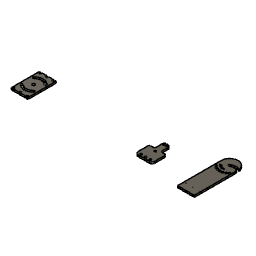
FS40 Pivot Bracket v27 (Autodesk Fusion 360 design; units mm, degrees)
Autodesk Fusion 360 part; units mm, degrees
note: some values were not read from the file. Set by a fixed rule: which sketch regions a step uses.
sketch "Schizzo5" plane through (0, 0, 0) normal (0, 0, 1) x (1, 0, 0)
  line L0 (484.2306, 82.5145) -> (484.2306, 12.5145)
  line L1 (463.4606, 82.5145) -> (463.4606, 12.5145) construction
  circle A0 centre (472.9306, 18.2645) radius 1.5
  line L2 (434.2306, 82.5145) -> (484.2306, 82.5145)
  line L3 (434.2306, 12.5145) -> (434.2306, 82.5145)
  line L4 (434.2306, 77.5145) -> (484.2306, 77.5145) construction
  circle A1 centre (463.4606, 77.5145) radius 1.5
  line L5 (472.9306, 82.5145) -> (472.9306, 12.5145) construction
  line L6 (484.2306, 12.5145) -> (434.2306, 12.5145)
  line L7 (434.2306, 18.2645) -> (484.2306, 18.2645) construction
  circle A2 centre (472.9306, 18.2645) radius 3
  circle A3 centre (463.4606, 77.5145) radius 3
  line L8 (434.2306, 47.2645) -> (484.2306, 47.2645) construction
  circle A4 centre (459.2306, 47.2645) radius 2.9
  line L9 (459.2306, 82.5145) -> (459.2306, 12.5145) construction
  circle A5 centre (459.2306, 47.2645) radius 29 construction
  line L10 (459.2306, 47.2645) -> (485, 47.2645) construction
  line L11 (459.2306, 47.2645) -> (485, 47.2645) construction
  line L12 (459.2306, 47.2645) -> (485, 47.2645) construction
  line L13 (459.2306, 47.2645) -> (485, 47.2645) construction
  circle A6 centre (459.2306, 18.2645) radius 2.9
  line L14 (631.2003, 146.4583) -> (631.2003, -8.5417)
  line L15 (581.2003, -8.5417) -> (581.2003, 146.4583)
  line L16 (631.2003, -8.5417) -> (581.2003, -8.5417)
  line L17 (610.4303, 146.4583) -> (610.4303, -8.5417) construction
  line L18 (581.2003, 146.4583) -> (631.2003, 146.4583)
  line L19 (619.9003, 146.4583) -> (619.9003, 0) construction
  line L20 (581.2003, 92.4583) -> (631.2003, 92.4583) construction
  circle A7 centre (619.9003, 92.4583) radius 1.6 construction
  line L21 (581.2003, 121.4583) -> (631.2003, 121.4583) construction
  line L22 (606.2003, 146.4583) -> (606.2003, 92.4583) construction
  circle A8 centre (606.2003, 121.4583) radius 3
  circle A9 centre (455.0006, 77.5145) radius 3
  circle A10 centre (455.0006, 77.5145) radius 1.5
  circle A11 centre (445.5306, 18.2645) radius 3
  circle A12 centre (445.5306, 18.2645) radius 1.5
  line L23 (581.2003, 96.4583) -> (631.2003, 96.4583) construction
  circle A13 centre (732, 5) radius 4
  line L24 (722, 15) -> (742, 15)
  line L25 (742, 15) -> (742, -5)
  line L26 (742, -5) -> (722, -5)
  line L27 (722, -5) -> (722, 15)
  line L28 (732, 15) -> (732, -5) construction
  line L29 (722, 5) -> (742, 5) construction
  line L30 (765, 15) -> (785, 15)
  line L31 (785, 15) -> (785, -5)
  line L32 (785, -5) -> (765, -5)
  line L33 (765, -5) -> (765, 15)
  line L34 (775, 15) -> (775, -5) construction
  line L35 (765, 5) -> (785, 5) construction
  circle A14 centre (775, 5) radius 4.05
  line L36 (606.2003, 121.4583) -> (635.9708, 121.4583) construction
  line L37 (628.1133, 97.0484) -> (631.2003, 95.2658)
  circle A15 centre (606.2003, 121.4583) radius 25
  line L38 (606.2003, 121.4583) -> (615.5972, 124.8785)
  line L39 (606.2003, 121.4583) -> (612.6158, 121.4583) construction
  line L40 (615.5972, 124.8785) -> (623.5972, 124.8785)
  line L41 (623.5972, 124.8785) -> (631.2003, 120.4889)
  line L42 (623.5972, 124.8785) -> (631.2003, 124.8785) construction
  line L43 (607.2263, 118.6393) -> (616.1262, 121.8785)
  line L44 (616.1262, 121.8785) -> (622.7934, 121.8785)
  line L45 (622.7934, 121.8785) -> (629.7003, 117.8908)
  line L46 (605.1742, 124.2774) -> (615.0682, 127.8785)
  line L47 (615.0682, 127.8785) -> (624.401, 127.8785)
  line L48 (624.401, 127.8785) -> (632.7003, 123.087)
  line L49 (629.7003, 117.8908) -> (631.2003, 117.0248)
  line L50 (629.7003, 117.8908) -> (635.1005, 117.8908) construction
  line L51 (606.2003, 121.4583) -> (598.6947, 93.4465) construction
  line L52 (606.2003, 121.4583) -> (631.0591, 121.4583) construction
  line L53 (606.2003, 121.4583) -> (629.1613, 121.4583) construction
  circle A16 centre (609.0194, 122.4844) radius 3
  circle A17 centre (476.2306, 20.5145) radius 8
  circle A18 centre (442.2306, 20.5145) radius 8
  circle A19 centre (455.0006, 77.5145) radius 5
  circle A20 centre (463.4606, 77.5145) radius 5
  line L54 (450.0006, 82.5145) -> (450.0006, 33) construction
  line L55 (434.2306, 50.1645) -> (484.2306, 50.1645) construction
  circle A21 centre (438.2296, 50.1645) radius 4
  line L56 (434.2306, 54.1645) -> (484.2306, 54.1645) construction
  circle A22 centre (446.0006, 58.1645) radius 4
  line L57 (450.0006, 77.5145) -> (450.0006, 58.1645)
  line L58 (468.4606, 77.5145) -> (468.4606, 58.1645)
  circle A23 centre (472.4606, 58.1645) radius 4
  circle A24 centre (480.2317, 50.1645) radius 4
  line L59 (438.2296, 54.1645) -> (446.0006, 54.1645)
  line L60 (480.2317, 54.1645) -> (472.4606, 54.1645)
  line L61 (606.2003, 121.4583) -> (591.7004, 96.3435) construction
  line L62 (606.2003, 121.4583) -> (625.9829, 121.4583) construction
  line L63 (606.2003, 121.4583) -> (585.6943, 100.9521) construction
  line L64 (606.2003, 121.4583) -> (623.662, 121.4583) construction
  line L65 (606.2003, 121.4583) -> (627.0131, 121.4583) construction
  line L66 (605.0102, 102.4865) -> (609.02, 102.527) construction
  line L67 (609.02, 102.527) -> (608.9899, 105.5135) construction
  line L68 (608.9899, 105.5135) -> (604.98, 105.473) construction
  line L69 (604.98, 105.473) -> (605.0102, 102.4865) construction
  line L70 (609.6489, 101.3799) -> (612.6489, 101.3799) construction
  line L71 (612.6489, 101.3799) -> (612.6489, 105.3799) construction
  line L72 (612.6489, 105.3799) -> (609.6489, 105.3799) construction
  line L73 (609.6489, 105.3799) -> (609.6489, 101.3799) construction
  line L74 (615.0517, 103.2642) -> (619.0517, 103.2642) construction
  line L75 (619.0517, 103.2642) -> (619.0517, 108.2642) construction
  line L76 (619.0517, 108.2642) -> (615.0517, 108.2642) construction
  line L77 (615.0517, 108.2642) -> (615.0517, 103.2642) construction
  line L78 (619.5121, 109.488) -> (622.5272, 109.5277) construction
  line L79 (622.5272, 109.5277) -> (622.4879, 112.512) construction
  line L80 (622.4879, 112.512) -> (619.4728, 112.4723) construction
  line L81 (619.4728, 112.4723) -> (619.5121, 109.488) construction
  line L82 (80.7173, 80.3147) -> (80.7173, -3.6853)
  circle A25 centre (85.7173, -1.1853) radius 1.5
  circle A26 centre (105.7173, 38.3147) radius 25 construction
  arc A27 (125.5163, 58.1137) -> (105.7173, 66.3147) centre (105.7173, 38.3147) ccw
  circle A28 centre (123.395, 55.9924) radius 3
  circle A29 centre (88.0397, 55.9924) radius 3
  arc A30 (105.7173, 66.3147) -> (85.9183, 58.1137) centre (105.7173, 38.3147) ccw
  circle A31 centre (125.7173, 77.8147) radius 3
  arc A32 (105.7173, 10.3147) -> (125.5163, 18.5157) centre (105.7173, 38.3147) ccw
  line L83 (80.7173, 38.3147) -> (130.7173, 38.3147) construction
  circle A33 centre (105.7173, 77.8147) radius 1.5
  circle A34 centre (85.7173, 77.8147) radius 3
  line L84 (105.7173, 38.3147) -> (123.395, 20.6371) construction
  arc A35 (105.7173, 66.3147) -> (85.9183, 58.1137) centre (105.7173, 38.3147) ccw
  circle A36 centre (85.7173, 77.8147) radius 1.5
  line L85 (130.7173, 80.3147) -> (80.7173, 80.3147)
  arc A37 (125.5163, 58.1137) -> (105.7173, 66.3147) centre (105.7173, 38.3147) ccw
  circle A38 centre (125.7173, 77.8147) radius 1.5
  line L86 (105.7173, 38.3147) -> (89.6274, 54.4047) construction
  circle A39 centre (105.7173, 77.8147) radius 3
  arc A40 (105.7173, 10.3147) -> (125.5163, 18.5157) centre (105.7173, 38.3147) ccw
  line L87 (105.7173, 38.3147) -> (105.7173, 13.3147) construction
  circle A41 centre (105.7173, 38.3147) radius 4
  circle A42 centre (105.7173, -1.1853) radius 1.5
  circle A43 centre (88.0397, 20.6371) radius 3
  line L88 (130.7173, -3.6853) -> (130.7173, 80.3147)
  arc A44 (85.9183, 18.5157) -> (105.7173, 10.3147) centre (105.7173, 38.3147) ccw
  line L89 (85.7173, 80.3147) -> (85.7173, -3.6853) construction
  arc A45 (105.7173, 13.3147) -> (123.395, 20.6371) centre (105.7173, 38.3147) ccw
  circle A46 centre (123.395, 20.6371) radius 3
  circle A47 centre (85.7173, -1.1853) radius 3
  circle A48 centre (105.7173, -1.1853) radius 3
  circle A49 centre (125.7173, -1.1853) radius 1.5
  line L90 (105.7173, 38.3147) -> (123.668, 56.2654) construction
  line L91 (80.7173, -3.6853) -> (130.7173, -3.6853)
  circle A50 centre (125.7173, -1.1853) radius 3
  line L92 (80.7173, -1.1853) -> (130.7173, -1.1853) construction
  line L93 (105.7173, 38.3147) -> (88.0397, 20.6371) construction
  arc A51 (85.9183, 18.5157) -> (105.7173, 10.3147) centre (105.7173, 38.3147) ccw
  line L94 (105.7173, 80.3147) -> (105.7173, -3.6853) construction
  arc A52 (88.0397, 20.6371) -> (105.7173, 13.3147) centre (105.7173, 38.3147) ccw
  line L95 (105.7173, 38.3147) -> (105.7173, 63.3147) construction
  line L96 (105.7173, 38.3147) -> (105.7173, 63.3147) construction
  line L97 (105.7173, 38.3147) -> (105.7173, 13.3147) construction
  circle A53 centre (606.2003, 121.4583) radius 29 construction
  line L98 (606.2003, 121.4583) -> (606.2003, 92.4583) construction
  circle A54 centre (585.6943, 100.9521) radius 3
  circle A55 centre (591.7004, 96.3435) radius 3
  circle A56 centre (598.6947, 93.4465) radius 3
  circle A57 centre (606.2003, 92.4583) radius 3
  circle A58 centre (613.7059, 93.4465) radius 3
  circle A59 centre (620.7001, 96.3435) radius 3
  circle A60 centre (626.7062, 100.9521) radius 3
  circle A61 centre (619.9003, 92.4583) radius 3 construction
  arc A62 (105.7173, 16.3147) -> (121.2737, 22.7584) centre (105.7173, 38.3147) ccw
  arc A63 (90.161, 22.7584) -> (105.7173, 16.3147) centre (105.7173, 38.3147) ccw
  arc A64 (105.7173, 60.3147) -> (90.161, 53.8711) centre (105.7173, 38.3147) ccw
  arc A65 (121.2737, 53.8711) -> (105.7173, 60.3147) centre (105.7173, 38.3147) ccw
  dimension "d70" = 50
  dimension "d71" = 70
  dimension "d72" = 29.23
  dimension "d73" = 38.7
  dimension "d74" = 59.25
  dimension "d75" = 5
  dimension "d76" = 3
  dimension "d77" = 3
  dimension "d78" = 6
  dimension "d79" = 6
  dimension "d84" = 29
  dimension "d85" = 5.8
  dimension "d103" = 5.8
  dimension "d110" = 50
  dimension "d111" = 155
  dimension "d112" = 29.23
  dimension "d113" = 38.7
  dimension "d117" = 3.2
  dimension "d119" = 29
  dimension "d120" = 6
  dimension "d129" = 6
  dimension "d130" = 3
  dimension "d131" = 29.23
  dimension "d132" = 6
  dimension "d133" = 3
  dimension "d135" = 38.7
  dimension "d137" = 25
  dimension "d139" = 8
  dimension "d145" = 20
  dimension "d146" = 20
  dimension "d152" = 20
  dimension "d153" = 20
  dimension "d154" = 8.1
  dimension "d168" = 20
  dimension "d169" = 8
  dimension "d170" = 30
  dimension "d175" = 10
  dimension "d176" = 3
  dimension "d177" = -3
  dimension "d178" = 30
  dimension "d187" = 8
  dimension "d188" = 8
  dimension "d189" = 4
  dimension "d196" = 15
  dimension "d197" = 15
  dimension "d198" = 15
  dimension "d202" = 130
  dimension "d212" = 3
  dimension "d215" = 3
  dimension "d216" = 3
  dimension "d217" = 3
  dimension "d219" = 3
  dimension "d220" = 3
  dimension "d221" = 50
  dimension "d222" = 84
  dimension "d223" = 2.5
  dimension "d224" = 20
  dimension "d225" = 3
  dimension "d226" = 6
  dimension "d227" = 3
  dimension "d228" = 6
  dimension "d229" = 8
  dimension "d230" = 45
  dimension "d231" = 6
  dimension "d232" = 45
  dimension "d233" = 6
  dimension "d238" = 58
  dimension "d239" = 6
  dimension "d240" = 6
  dimension "d241" = 6
  dimension "d242" = 6
  dimension "d243" = 6
  dimension "d245" = 58
  dimension "d246" = -3
  dimension "d247" = -3
  text T0 "0°" font "Arial" height 3 align left top in box 4.01 x 2.9866 at (605.0102, 102.4865) x (0.999949, 0.010082) y (-0.010082, 0.999949) spacing 1
  text T1 "15°" font "Arial" height 3 align left top in box 3 x 4 at (609.6489, 101.3799) x (1, 0) y (0, 1) spacing 1
  text T2 "30°" font "Arial" height 3 align left top in box 4 x 5 at (615.0517, 103.2642) x (1, 0) y (0, 1) spacing 1
  text T3 "45°" font "Arial" height 3 align left top in box 3.0153 x 2.9846 at (619.5121, 109.488) x (0.999913, 0.01317) y (-0.01317, 0.999913) spacing 1
  constraint horizontal L6
  constraint vertical L3
  constraint horizontal L2
  constraint vertical L0
  constraint coincident L1.start L2
  constraint coincident L1.end L6
  constraint perpendicular L1 L6
  constraint coincident L5.start L2
  constraint perpendicular L2 L5
  constraint coincident L4.start L3
  constraint coincident L4.end L0
  constraint perpendicular L0 L4
  constraint coincident L7.start L3
  constraint coincident L7.end L0
  constraint perpendicular L0 L7
  constraint coincident A1.centre L1
  constraint coincident A1.centre L4
  constraint coincident A0.centre L5
  constraint coincident A0.centre L7
  constraint concentric A0 A2
  constraint concentric A1 A3
  constraint coincident L3 L8.start
  constraint coincident L0 L8.end
  constraint perpendicular L0 L8
  constraint midpoint L2 L9.start
  constraint midpoint L6 L9.end
  constraint coincident A4.centre L9
  constraint coincident L8 A4.centre
  constraint concentric A4 A5
  constraint horizontal L10
  constraint coincident A4.centre A5.centre
  constraint horizontal L11
  constraint horizontal L12
  constraint horizontal L13
  constraint coincident A5 A6.centre
  constraint coincident L9 A6.centre
  constraint horizontal L16
  constraint vertical L15
  constraint horizontal L18
  constraint vertical L14
  constraint coincident L17.start L18
  constraint coincident L17.end L16
  constraint perpendicular L16 L17
  constraint coincident L19.start L18
  constraint perpendicular L18 L19
  constraint coincident L20.start L15
  constraint coincident L20.end L14
  constraint perpendicular L14 L20
  constraint coincident A7.centre L19
  constraint coincident A7.centre L20
  constraint coincident L15 L21.start
  constraint coincident L14 L21.end
  constraint perpendicular L14 L21
  constraint midpoint L18 L22.start
  constraint midpoint L20 L22.end
  constraint midpoint L21 A8.centre
  constraint coincident L4 A9.centre
  constraint concentric A9 A10
  constraint coincident L7 A11.centre
  constraint concentric A11 A12
  constraint coincident L15 L23.start
  constraint coincident L14 L23.end
  constraint perpendicular L14 L23
  constraint horizontal L24
  constraint vertical L25
  constraint horizontal L26
  constraint vertical L27
  constraint midpoint L24 L28.start
  constraint midpoint L26 L28.end
  constraint midpoint L27 L29.start
  constraint midpoint L25 L29.end
  constraint coincident A13.centre L28
  constraint coincident A13.centre L29
  constraint horizontal L30
  constraint vertical L31
  constraint horizontal L32
  constraint vertical L33
  constraint midpoint L30 L34.start
  constraint midpoint L32 L34.end
  constraint midpoint L33 L35.start
  constraint midpoint L31 L35.end
  constraint midpoint L34 A14.centre
  constraint horizontal L36
  constraint coincident A8.centre L36.start
  constraint coincident L14 L37.end
  constraint tangent L15 A15
  constraint tangent L18 A15
  constraint tangent L14 A15
  constraint horizontal L39
  constraint horizontal L40
  constraint horizontal L42
  constraint coincident L14 L41.end
  constraint horizontal L50
  constraint coincident L14 L49.end
  constraint horizontal L52
  constraint horizontal L53
  constraint coincident A8 A16.centre
  constraint coincident L38 A16.centre
  constraint coincident A8.centre A16
  constraint coincident L14 L42.end
  constraint tangent L6 A17
  constraint tangent L0 A17
  constraint symmetric L9 A17 A18
  constraint concentric A9 A19
  constraint tangent L2 A19
  constraint symmetric L9 A19 A20
  constraint coincident L2 L54.start
  constraint perpendicular L8 L54
  constraint tangent A19 L54
  constraint coincident L3 L55.start
  constraint coincident L0 L55.end
  constraint perpendicular L0 L55
  constraint tangent A4 L55
  constraint coincident L55 A21.centre
  constraint coincident L3 L56.start
  constraint coincident L0 L56.end
  constraint perpendicular L0 L56
  constraint tangent A21 L56
  constraint tangent L56 A22
  constraint tangent L54 A22
  constraint coincident A19 L57.start
  constraint coincident A22 L57.end
  constraint coincident L54 L57.end
  constraint symmetric L9 A21 A24
  constraint symmetric L9 A22 A23
  constraint symmetric L9 L57.start L58.start
  constraint symmetric L9 L57.end L58.end
  constraint coincident L56 L59.start
  constraint coincident A21 L59.start
  constraint coincident A22 L59.end
  constraint coincident L56 L59.end
  constraint symmetric L9 L59.start L60.start
  constraint symmetric L9 L59.end L60.end
  constraint tangent A19 L57
  constraint horizontal L62
  constraint horizontal L64
  constraint horizontal L65
  constraint coincident L5.end L6
  constraint horizontal L91
  constraint vertical L88
  constraint horizontal L85
  constraint vertical L82
  constraint midpoint L94.start L85
  constraint midpoint L94.end L91
  constraint coincident L92.end L88
  constraint perpendicular L88 L92
  constraint midpoint L83.start L82
  constraint midpoint L83.end L88
  constraint coincident L89.start L85
  constraint coincident L89.end L91
  constraint perpendicular L89 L91
  constraint coincident A25.centre L92
  constraint coincident A25.centre L89
  constraint concentric A25 A47
  constraint symmetric A25 A49 L94
  constraint symmetric A47 A50 L94
  constraint symmetric A25 L83 A36
  constraint symmetric L83 A34 A47
  constraint symmetric L83 A38 A49
  constraint symmetric A31 L83 A50
  constraint coincident A42.centre L94
  constraint coincident A42.centre L92
  constraint concentric A42 A48
  constraint symmetric L83 A33 A42
  constraint symmetric L83 A39 A48
  constraint midpoint A26.centre L83
  constraint concentric A26 A41
  constraint tangent A26 L88
  constraint coincident L87.end A26
  constraint coincident L87.end L94
  constraint coincident A26.centre A27.centre
  constraint coincident A43.centre L93.end
  constraint coincident L84.end A45.end
  constraint coincident L95.end A26
  constraint coincident L95.end L94
  constraint symmetric A29 L83 A43
  constraint symmetric A28 L83 A46
  constraint symmetric A32.start A27.end L83
  constraint symmetric A44.start A30.end L83
  constraint symmetric A30 L83 A44
  constraint symmetric A32.end A27.start L83
  constraint symmetric A27 L83 A40
  constraint symmetric A30.end A44.start L83
  constraint symmetric L83 A35 A51
  constraint symmetric A32 L83 A37
  constraint coincident L63.end A53
  constraint coincident A53 L22.end
  constraint perpendicular L52 L98
  constraint coincident L61.end A53
  constraint coincident L51.end A53
  constraint coincident L63.end A54.centre
  constraint coincident L61.end A55.centre
  constraint coincident L51.end A56.centre
  constraint coincident L22.end L98.end
  constraint symmetric L98 A54 A60
  constraint symmetric L98 A55 A59
  constraint symmetric L98 A56 A58
  constraint concentric A7 A61
  constraint symmetric L83 A62.end A65.start
  constraint symmetric L83 A62.start A64.start
  constraint symmetric L83 A62 A65
  constraint symmetric L83 A63.start A64.end
  constraint symmetric L83 A63 A64
  constraint coincident L92.start L82
  measures "d70" distance of L3.start L0.end
  measures "d71" distance of L0.end L0.start
  measures "d72" distance of L1 L3
  measures "d73" distance of L3 L5
  measures "d74" distance of L4 L7
  measures "d75" distance of L2 L4
  measures "d76" diameter of A1
  measures "d77" diameter of A0
  measures "d78" diameter of A2
  measures "d79" diameter of A3
  measures "d84" distance of L7 L8
  measures "d85" diameter of A4
  measures "d103" diameter of A6
  measures "d110" distance of L14.end L15.start
  measures "d111" distance of L14.end L14.start
  measures "d112" distance of L15 L17
  measures "d113" distance of L15 L19
  measures "d117" diameter of A7
  measures "d119" distance of L20 L21
  measures "d120" diameter of A8
  measures "d129" diameter of A9
  measures "d130" diameter of A10
  measures "d131" distance of L0 A9.centre
  measures "d132" diameter of A11
  measures "d133" diameter of A12
  measures "d135" distance of L0 A11.centre
  measures "d137" distance of L21 L23
  measures "d139" diameter of A13
  measures "d145" distance of L24.start L24.end
  measures "d146" distance of L24.start L26.end
  measures "d152" distance of L30.start L30.end
  measures "d153" distance of L30.start L32.end
  measures "d154" diameter of A14
  measures "d168" angle of L38 L39
  measures "d169" distance of L38.end L40.end
  measures "d170" angle of L41 L42
  measures "d175" distance of A8.centre L38.end
  measures "d178" angle of L49 L50
  measures "d187" radius of A17
  measures "d188" diameter of A21
  measures "d189" radius of A22
  measures "d196" angle of L61 L63
  measures "d197" angle of L51 L61
  measures "d198" angle of L22 L51
  measures "d202" distance of L16 L21
  measures "d221" distance of L82.end L88.start
  measures "d222" distance of L82.end L82.start
  measures "d223" distance of L91 L92
  measures "d224" distance of L89 L94
  measures "d225" diameter of A25
  measures "d226" diameter of A47
  measures "d227" diameter of A42
  measures "d228" diameter of A48
  measures "d229" diameter of A41
  measures "d230" angle of L93 L97
  measures "d231" diameter of A43
  measures "d232" angle of L84 L87
  measures "d233" diameter of A46
  measures "d238" diameter of A53
  measures "d239" diameter of A54
  measures "d240" diameter of A55
  measures "d241" diameter of A56
  measures "d242" diameter of A57
  measures "d243" diameter of A61
  measures "d245" diameter of A5
extrude "Estrusione12" add sketch "Schizzo5" along normal blind 5 contours A24 | L0 L3 L6 A17 A18 A19 A20 A21 A22 L57 L58 A23 A24 L59 L60 | L2 A19 A20 | A19 A20 | A17 | A19 A20 | A19 A20 | A18 | A21 makes body 1
extrude "Estrusione13" add sketch "Schizzo5" along normal blind 1.8 contours A2 | A3 | A9 | A11 bodies 1
extrude "Estrusione24" add sketch "Schizzo5" along normal blind 5 separate body contours L82 A31 A34 L85 A39 L88 A47 A48 L91 A50 makes body 2
extrude "Estrusione25" add sketch "Schizzo5" along normal blind 1.8 contours A34 L85 | A47 L91 | L85 A39 | A48 L91 | A31 L85 | L91 A50 picked at (85.7547, 79.98) picked at (85.7547, -3.3505) picked at (105.7547, 79.98) picked at (105.7547, -3.3505) picked at (125.7547, 79.98) picked at (125.7547, -3.3505) bodies 2
extrude "Estrusione15" add sketch "Schizzo5" along normal blind 5 separate body contours A8 A15 L43 L44 L45 L46 L47 L48 L49 | L14 L15 L16 A15 L49 | A8 L46 A16 | A8 L43 A16 makes body 3
sketch "Foratura Spalla" plane through (0, -8.5417, 0) normal (0, -1, 0) x (1, 0, 0)
  line L0 (581.2003, 0) -> (631.2003, 0)
  line L1 (631.2003, 0) -> (631.2003, 5)
  line L2 (631.2003, 5) -> (581.2003, 5)
  line L3 (581.2003, 5) -> (581.2003, 0)
  line L4 (581.2003, 2.5) -> (631.2003, 2.5) construction
  line L5 (606.2003, 5) -> (606.2003, 0) construction
  circle A0 centre (606.2003, 2.5) radius 1.4
  line L6 (586.2003, 0) -> (586.2003, 5) construction
  circle A1 centre (586.2003, 2.5) radius 1.4
  circle A2 centre (626.2003, 2.5) radius 1.4
  dimension "d124" = 2.8
  dimension "d125" = 20
  dimension "d126" = 2.8
  constraint midpoint L3 L4.start
  constraint midpoint L1 L4.end
  constraint midpoint L2 L5.start
  constraint midpoint L0 L5.end
  constraint midpoint L5 A0.centre
  constraint coincident L0 L6.start
  constraint coincident L2 L6.end
  constraint perpendicular L2 L6
  constraint midpoint L6 A1.centre
  constraint symmetric L5 A1 A2
  measures "d124" diameter of A0
  measures "d125" distance of A0.centre L6
  measures "d126" diameter of A1
extrude "Estrusione16" cut sketch "Foratura Spalla" against normal blind 20 contours A0 | A1 | A2 bodies 3
extrude "Estrusione17" add sketch "Schizzo5" along normal blind 5 separate body contours A13 makes body 4
sketch "Schizzo15" plane through (0, 0, 5) normal (0, 0, 1) x (-1, 0, 0)
  line L0 (-607.9933, -125.3035) -> (-615.0682, -127.8785)
  line L1 (-615.0682, -127.8785) -> (-624.401, -127.8785)
  line L2 (-624.401, -127.8785) -> (-631.0677, -124.0296)
  arc A0 (-631.0677, -124.0296) -> (-581.2003, -121.4583) centre (-606.2003, -121.4583) ccw
  line L3 (-581.2003, -121.4583) -> (-581.2003, 8.5417)
  line L4 (-581.2003, 8.5417) -> (-631.2003, 8.5417)
  line L5 (-631.2003, 8.5417) -> (-631.2003, -117.0248)
  line L6 (-631.2003, -117.0248) -> (-622.7934, -121.8785)
  line L7 (-622.7934, -121.8785) -> (-616.1262, -121.8785)
  line L8 (-616.1262, -121.8785) -> (-610.0454, -119.6653)
  arc A1 (-608.4984, -119.53) -> (-610.0454, -119.6653) centre (-609.0194, -122.4844) ccw
  arc A2 (-606.7212, -124.4128) -> (-608.4984, -119.53) centre (-606.2003, -121.4583) ccw
  arc A3 (-607.9933, -125.3035) -> (-606.7212, -124.4128) centre (-609.0194, -122.4844) ccw
  line L9 (-604.6879, -101.2309) -> (-607.7132, -101.231) construction
  line L10 (-607.7132, -101.231) -> (-607.713, -104.9906) construction
  line L11 (-607.713, -104.9906) -> (-604.6877, -104.9904) construction
  line L12 (-604.6877, -104.9904) -> (-604.6879, -101.2309) construction
  line L13 (-599, -102) -> (-602, -102) construction
  line L14 (-602, -102) -> (-602, -105) construction
  line L15 (-602, -105) -> (-599, -105) construction
  line L16 (-599, -105) -> (-599, -102) construction
  line L17 (-594, -103.5) -> (-597.7138, -103.5) construction
  line L18 (-597.7138, -103.5) -> (-597.7138, -107) construction
  line L19 (-597.7138, -107) -> (-594, -107) construction
  line L20 (-594, -107) -> (-594, -103.5) construction
  line L21 (-589.0011, -106.9973) -> (-594, -107) construction
  line L22 (-594, -107) -> (-593.9979, -111.0053) construction
  line L23 (-593.9979, -111.0053) -> (-588.9989, -111.0027) construction
  line L24 (-588.9989, -111.0027) -> (-589.0011, -106.9973) construction
  circle A4 centre (-626.7062, -100.9521) radius 3
  circle A5 centre (-606.2003, -92.4583) radius 3
  circle A6 centre (-585.6943, -100.9521) radius 3
  circle A7 centre (-591.7004, -96.3435) radius 3
  circle A8 centre (-620.7001, -96.3435) radius 3
  circle A9 centre (-598.6947, -93.4465) radius 3
  circle A10 centre (-613.7059, -93.4465) radius 3
  dimension "d205" = 3
  dimension "d207" = 3
  dimension "d208" = 3
  dimension "d209" = 3
  text T0 "0°" font "Arial" height 3 align left top in box 3.0253 x 3.7596 at (-604.6879, -101.2309) x (-1, -0.000046) y (0.000046, -1) spacing 1
  text T1 "15°" font "Arial" height 3 align left top in box 3 x 3 at (-599, -102) x (-1, 0) y (0, -1) spacing 1
  text T2 "30°" font "Arial" height 3 align left top in box 3.7138 x 3.5 at (-594, -103.5) x (-1, 0) y (0, -1) spacing 1
  text T3 "45°" font "Arial" height 3 align left top in box 4.9989 x 4.0053 at (-589.0011, -106.9973) x (-1, -0.000533) y (0.000533, -1) spacing 1
extrude "Estrusione22" cut sketch "Schizzo15" against normal blind 1 text T3 T2 T1 T0 bodies 3
extrude "Estrusione23" cut sketch "Schizzo5" along normal blind 1 text T0 T1 T2 T3 bodies 3
sketch "Schizzo9" plane through (0, 0, 0) normal (0, 0, 1) x (1, 0, 0)
extrude "Estrusione18" add sketch "Schizzo5" against normal blind 5 contours A13 | L24 L25 L26 L27 bodies 4
ref_plane "Piano di lavoro2" through (728.0171, 5.3698, 5) normal (-0.092451, -0.995717, 0) x (0.995717, -0.092451, 0)
sketch "Schizzo11" plane through (728.0171, 5.3698, 5) normal (-0.092451, -0.995717, 0) x (0.995717, -0.092451, 0)
  line L0 (0, 0) -> (8, 0) construction
  line L1 (8, 0) -> (8, -5) construction
  line L2 (8, -5) -> (0, -5) construction
  line L3 (0, -5) -> (0, 0) construction
  line L4 (0, -2.5) -> (8, -2.5) construction
  circle A0 centre (0, -2.5) radius 0.75
  dimension "d150" = 1.5
  constraint horizontal L0
  constraint vertical L1
  constraint horizontal L2
  constraint vertical L3
  constraint coincident L0.start L3.end
  constraint midpoint L3 L4.start
  constraint midpoint L1 L4.end
  constraint coincident L4.start A0.centre
  measures "d150" diameter of A0
revolve "Rivoluzione2" cut sketch "Schizzo11" angle 360 about axis through (732, 5, -2.5) along (0, 0, 1) bodies 4
extrude "Estrusione19" add sketch "Schizzo5" along normal blind 5 separate body contours L30 L31 L32 L33 makes body 5
ref_plane "Piano di lavoro3" through (775, 5, 2.5) normal (0, -1, 0) x (1, 0, 0)
sketch "Schizzo13" plane through (0, 5, 0) normal (0, -1, 0) x (1, 0, 0)
  line L0 (765, 0) -> (785, 0)
  line L1 (785, 0) -> (785, 5)
  line L2 (785, 5) -> (765, 5)
  line L3 (765, 5) -> (765, 0)
  line L4 (765, 2.5) -> (785, 2.5) construction
  line L5 (779.5, 0) -> (770.5, 0) construction
  line L6 (770.5, 0) -> (770.5, 5) construction
  line L7 (770.5, 5) -> (779.5, 5) construction
  line L8 (779.5, 5) -> (779.5, 0) construction
  line L9 (779.5, 0) -> (770.5, 5) construction
  line L10 (770.5, 0) -> (779.5, 5) construction
  line L11 (785, 0) -> (765, 0) construction
  circle A0 centre (770.5, 2.5) radius 0.8
  circle A1 centre (771.3, 2.5) radius 0.8
  line L12 (770.5, 3.3) -> (771.3, 3.3)
  line L13 (770.5, 1.7) -> (771.3, 1.7)
  point P0 (775, 2.5)
  dimension "d158" = 9
  dimension "d159" = 1.6
  constraint midpoint L3 L4.start
  constraint midpoint L1 L4.end
  constraint horizontal L5
  constraint perpendicular L5 L6
  constraint parallel L5 L7
  constraint parallel L6 L8
  constraint coincident L9 P0
  constraint coincident L10 P0
  constraint midpoint L4 P0
  constraint collinear L5 L11
  constraint midpoint L6 A0.centre
  constraint coincident A0 A1.centre
  constraint coincident L4 A1.centre
  constraint coincident A0.centre A1
  constraint coincident A0 L12.start
  constraint coincident L6 L12.start
  constraint coincident A1 L12.end
  constraint tangent A1 L12
  constraint coincident L6 L13.start
  constraint coincident A0 L13.start
  constraint coincident A1 L13.end
  constraint tangent A1 L13
  measures "d158" distance of L6.end L7.end
  measures "d159" diameter of A0
revolve "Rivoluzione3" cut sketch "Schizzo13" angle 360 about axis through (775, 5, -2.5) along (0, 0, 1) contours A0 A1 | A0 A1 L12 | A0 A1 L13 | A0 A1 | A0 A1 bodies 5
hidden bodies 4 5
equation "d103 = d85"
equation "d117 = d138"
equation "d138 = 3.2 mm"
equation "d176 = d120 / 2"
equation "d177 = -d120 / 2"
equation "d178 = d170"
equation "d225 = d227"
equation "d226 = d228"
equation "d239 = d120"
equation "d240 = d120"
equation "d241 = d120"
equation "d242 = d120"
named bodies: "Spalla Perno", "Adattatore", "Base"
